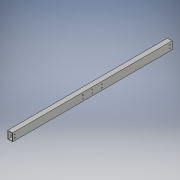
# Autodesk Inventor part: 前後機構_角柱1
Saved by Autodesk Inventor 2019.4 (Build 234330000, 330)
## iProperties
Created: 2021-12-05
Part Number: 前後機構_角柱1
Material: アルミニウム 6061
Document SubType Name: Modeling
Designer: 堀川皓史
Density: 2.7 g/cm^3
Appearance: アルミニウム - フラット
Author: 堀川皓史
Autodesk Inventor part; units mm, degrees
ref_plane "YZ Plane" through (0, 0, 0) normal (1, 0, 0) x (0, 1, 0)
ref_plane "XZ Plane" through (0, 0, 0) normal (0, 1, 0) x (-1, 0, 0)
ref_plane "XY Plane" through (0, 0, 0) normal (0, 0, 1) x (1, 0, 0)
sketch "スケッチ1" plane through (0, 0, 0) normal (0, 0, 1) x (1, 0, 0)
  line L0 (7.5, 12.5) -> (-7.5, 12.5)
  line L1 (-7.5, 12.5) -> (-7.5, -12.5)
  line L2 (-7.5, -12.5) -> (7.5, -12.5)
  line L3 (7.5, -12.5) -> (7.5, 12.5)
  line L4 (7.5, 12.5) -> (-7.5, -12.5) construction
  line L5 (-7.5, 12.5) -> (7.5, -12.5) construction
  line L6 (-5.5, 10.5) -> (5.5, 10.5)
  line L7 (5.5, 10.5) -> (5.5, -10.5)
  line L8 (5.5, -10.5) -> (-5.5, -10.5)
  line L9 (-5.5, -10.5) -> (-5.5, 10.5)
  point P0 (0, 0)
  dimension "d0" = 15
  dimension "d1" = 25
  dimension "d2" = 2
  constraints: 20 end point, 4 parallel, 2 midpoint, 2 perpendicular, 1 horizontal, 3 other
  measures "d0" distance of L2.end L1.end
  measures "d1" distance of L1.end L0.end
  measures "d2" distance between parallel lines of L0 L6
extrude "押し出し1" add sketch "スケッチ1" along normal blind 512
sketch "スケッチ2" plane through (7.5, -12.5, 0) normal (1, 0, 0) x (0, 0, -1)
  circle A0 centre (-7, 17.5) radius 1.6
  circle A1 centre (-7, 7.5) radius 1.6
  circle A2 centre (-505, 17.5) radius 1.6
  circle A3 centre (-505, 7.5) radius 1.6
  line L0 (-512, 0) -> (-512, 25) projected
  line L1 (0, 25) -> (-512, 25) projected
  line L2 (0, 0) -> (-512, 0) projected
  line L3 (0, 0) -> (0, 25) projected
  circle A4 centre (-256, 17.5) radius 1.6
  circle A5 centre (-286, 17.5) radius 1.6
  circle A6 centre (-226, 17.5) radius 1.6
  circle A7 centre (-256, 7.5) radius 1.6
  circle A8 centre (-286, 7.5) radius 1.6
  circle A9 centre (-226, 7.5) radius 1.6
  line L4 (-226, 17.5) -> (-286, 17.5) construction
  line L5 (-286, 17.5) -> (-286, 7.5) construction
  line L6 (-286, 7.5) -> (-226, 7.5) construction
  line L7 (-226, 7.5) -> (-226, 17.5) construction
  line L8 (-226, 17.5) -> (-286, 7.5) construction
  line L9 (-286, 17.5) -> (-226, 7.5) construction
  point P0 (-256, 12.5)
  point P1 (-256, 17.5)
  point P2 (-256, 7.5)
  dimension "d7" = 3.2
  dimension "d8" = 3.2
  dimension "d13" = 3.2
  dimension "d14" = 3.2
  dimension "d17" = 10
  dimension "d23" = 7
  dimension "d24" = 7.5
  dimension "d25" = 10
  dimension "d26" = 7.5
  dimension "d27" = 7
  dimension "d28" = 3.2
  dimension "d29" = 3.2
  dimension "d30" = 3.2
  dimension "d31" = 3.2
  dimension "d32" = 3.2
  dimension "d33" = 3.2
  dimension "d34" = 60
  dimension "d35" = 10
  dimension "d36" = 256
  dimension "d37" = 7.5
  constraints: 12 end point, 10 centre point, 6 coincident, 4 midpoint, 2 parallel, 2 vertical alignment, 1 horizontal, 1 perpendicular
  measures "d7" diameter of A0
  measures "d8" diameter of A1
  measures "d13" diameter of A2
  measures "d14" diameter of A3
  measures "d17" distance of A3.centre A2.centre
  measures "d23" distance from line of L0 A3.centre
  measures "d24" distance from line of L2 A3.centre
  measures "d25" distance of A1.centre A0.centre
  measures "d26" distance from line of L2 A1.centre
  measures "d27" distance from line of L3 A1.centre
  measures "d28" diameter of A4
  measures "d29" diameter of A5
  measures "d30" diameter of A6
  measures "d31" diameter of A7
  measures "d32" diameter of A8
  measures "d33" diameter of A9
  measures "d34" distance of L6.end L5.end
  measures "d35" distance of L5.end L4.end
  measures "d36" distance from line of L3 point (-256, 12.5)
  measures "d37" distance between parallel lines of L4 L1
extrude "押し出し2" cut sketch "スケッチ2" against normal through all contours A0 | A1 | A2 | A3 | A4 | A5 | A6 | A7 | A8 | A9
